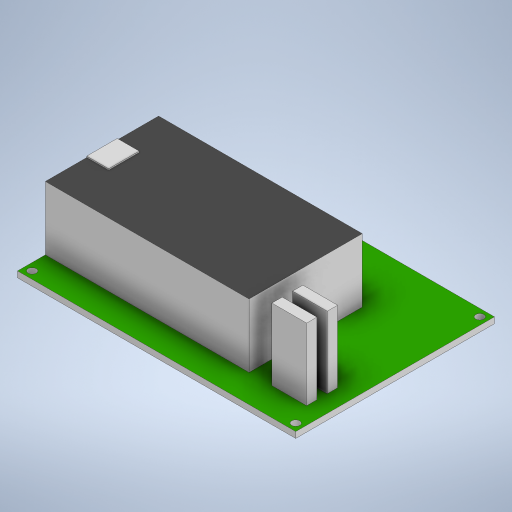
# Autodesk Inventor part: PCBModel
Saved by Autodesk Inventor 2024 (Build 280153000, 153)
## iProperties
Created: 2024-05-21
Part Number: PCBModel
Material: Generic
Document SubType Name: Modeling
Designer: andre
Density: 1 g/cm^3
Appearance: Default
Author: andre
Autodesk Inventor part; units mm, degrees
ref_plane "YZ Plane" through (0, 0, 0) normal (1, 0, 0) x (0, 1, 0)
ref_plane "XZ Plane" through (0, 0, 0) normal (0, 1, 0) x (-1, 0, 0)
ref_plane "XY Plane" through (0, 0, 0) normal (0, 0, 1) x (1, 0, 0)
sketch "Sketch1" plane through (0, 0, 0) normal (0, 1, 0) x (-1, 0, 0)
  line L0 (-35, 25) -> (35, 25)
  line L1 (35, 25) -> (35, -25)
  line L2 (35, -25) -> (-35, -25)
  line L3 (-35, -25) -> (-35, 25)
  line L4 (-35, 25) -> (35, -25) construction
  line L5 (35, 25) -> (-35, -25) construction
  point P0 (0, 0)
  dimension "d0" = 70
  dimension "d1" = 50
  constraints: 12 end point, 2 midpoint, 2 parallel, 1 horizontal, 1 perpendicular
  measures "d0" distance of L1.end L2.end
  measures "d1" distance of L0.end L1.end
extrude "Extrusion1" add sketch "Sketch1" along normal blind 1.5
sketch "Sketch4" plane through (0, 1.5, 0) normal (0, 1, 0) x (1, 0, 0)
  line L0 (16.25, 10.5) -> (-35, 10.5)
  line L1 (-35, 10.5) -> (-35, -18)
  line L2 (-35, -18) -> (16.25, -18)
  line L3 (16.25, -18) -> (16.25, 10.5)
  line L4 (16.25, 10.5) -> (-35, -18) construction
  line L5 (-35, 10.5) -> (16.25, -18) construction
  line L6 (-35, -25) -> (35, -25) projected
  line L7 (-35, 25) -> (-35, -25) projected
  dimension "d10" = 51.25
  dimension "d11" = 28.5
  dimension "d12" = 7
  constraints: 12 end point, 2 parallel, 1 collinear, 1 horizontal, 1 perpendicular
  measures "d10" distance of L2.end L1.end
  measures "d11" distance of L1.end L0.end
  measures "d12" distance between parallel lines of L6 L2
extrude "Extrusion3" add sketch "Sketch4" along normal blind 16
sketch "Sketch5" plane through (0, 1.5, 0) normal (0, 1, 0) x (1, 0, 0)
  line L0 (30.74, -15.4) -> (22, -15.4)
  line L1 (22, -15.4) -> (22, -18)
  line L2 (22, -18) -> (30.74, -18)
  line L3 (30.74, -18) -> (30.74, -15.4)
  line L4 (30.74, -15.4) -> (22, -18) construction
  line L5 (22, -15.4) -> (30.74, -18) construction
  line L6 (16.25, -18) -> (16.25, 10.5) projected
  line L7 (-35, -18) -> (16.25, -18) projected
  line L8 (30.74, -10.2) -> (22, -10.2)
  line L9 (22, -10.2) -> (22, -12.8)
  line L10 (22, -12.8) -> (30.74, -12.8)
  line L11 (30.74, -12.8) -> (30.74, -10.2)
  line L12 (30.74, -10.2) -> (22, -12.8) construction
  line L13 (22, -10.2) -> (30.74, -12.8) construction
  point P0 (0, 0)
  point P1 (26.37, -16.7)
  point P2 (22, -16.7)
  point P3 (26.37, -11.5)
  point P4 (22, -11.5)
  dimension "d15" = 5.75
  dimension "d16" = 8.74
  dimension "d17" = 2.6
  dimension "d18" = 8.74
  dimension "d19" = 2.6
  dimension "d20" = 2.6
  constraints: 24 end point, 6 midpoint, 4 parallel, 2 horizontal, 2 perpendicular, 1 collinear
  measures "d15" distance from line of L6 point (22, -16.7)
  measures "d16" distance of L1.end L2.end
  measures "d17" distance of L2.end L0.start
  measures "d18" distance of L9.end L10.end
  measures "d19" distance of L10.end L8.start
  measures "d20" distance between parallel lines of L0 L10
extrude "Extrusion4" add sketch "Sketch5" along normal blind 18
sketch "Sketch6" plane through (-35, 0, -25) normal (-1, 0, 0) x (0, 0, 1)
  line L0 (24.91, 17.82) -> (32.59, 17.82)
  line L1 (32.59, 17.82) -> (32.59, 15.11)
  line L2 (32.59, 15.11) -> (24.91, 15.11)
  line L3 (24.91, 15.11) -> (24.91, 17.82)
  line L4 (24.91, 17.82) -> (32.59, 15.11) construction
  line L5 (32.59, 17.82) -> (24.91, 15.11) construction
  line L6 (43, 1.5) -> (50, 1.5) projected
  line L7 (43, 1.5) -> (43, 17.5) projected
  line L8 (14.5, 1.5) -> (14.5, 17.5) projected
  line L9 (32.18, 17.41) -> (25.32, 17.41)
  line L10 (25.32, 17.41) -> (25.32, 15.52)
  line L11 (25.32, 15.52) -> (32.18, 15.52)
  line L12 (32.18, 15.52) -> (32.18, 17.41)
  point P0 (25, 0)
  point P1 (28.75, 16.465)
  dimension "d23" = 16.32
  dimension "d24" = 2.71
  dimension "d25" = 7.68
  dimension "d26" = 14.25
  dimension "d27" = 14.25
  dimension "d28" = 0.41
  constraints: 20 end point, 4 parallel, 2 midpoint, 2 perpendicular, 1 horizontal, 3 other
  measures "d23" distance between parallel lines of L6 L0
  measures "d24" distance between parallel lines of L0 L2
  measures "d25" distance between parallel lines of L3 L1
  measures "d26" distance from line of point (28.75, 16.465) L7
  measures "d27" distance from line of L8 point (28.75, 16.465)
  measures "d28" distance between parallel lines of L0 L9
extrude "Extrusion5" add sketch "Sketch6" against normal blind 5.51
sketch "Sketch7" plane through (-35, 0, -25) normal (-1, 0, 0) x (0, 0, 1)
  line L0 (32.18, 17.41) -> (25.32, 17.41) projected
  line L1 (25.32, 17.41) -> (25.32, 15.52) projected
  line L2 (25.32, 15.52) -> (32.18, 15.52) projected
  line L3 (32.18, 15.52) -> (32.18, 17.41) projected
  point P0 (25, 0)
extrude "Extrusion6" cut sketch "Sketch7" against normal blind 4.99
sketch "Sketch8" plane through (0, 1.5, 0) normal (0, 1, 0) x (1, 0, 0)
  circle A0 centre (33.16, -23.16) radius 1
  circle A1 centre (-33.16, -23.16) radius 1
  circle A2 centre (-33.16, 23.16) radius 1
  circle A3 centre (33.16, 23.16) radius 1
  line L0 (22, -10.2) -> (30.74, -10.2) projected
  line L1 (30.74, -10.2) -> (30.74, -12.8) projected
  line L2 (30.74, -12.8) -> (22, -12.8) projected
  line L3 (22, -12.8) -> (22, -10.2) projected
  line L4 (22, -15.4) -> (30.74, -15.4) projected
  line L5 (30.74, -15.4) -> (30.74, -18) projected
  line L6 (30.74, -18) -> (22, -18) projected
  line L7 (22, -18) -> (22, -15.4) projected
  line L8 (16.25, -18) -> (-35, -18) projected
  line L9 (-35, -18) -> (-35, -25) projected
  line L10 (-35, -25) -> (35, -25) projected
  line L11 (35, -25) -> (35, 25) projected
  line L12 (35, 25) -> (-35, 25) projected
  line L13 (-35, 25) -> (-35, 10.5) projected
  line L14 (-35, 10.5) -> (16.25, 10.5) projected
  line L15 (16.25, 10.5) -> (16.25, -18) projected
  point P0 (0, 0)
  dimension "d33" = 2
  dimension "d34" = 2
  dimension "d35" = 2
  dimension "d36" = 2
  dimension "d37" = 1.84
  dimension "d38" = 1.84
  dimension "d39" = 1.84
  dimension "d40" = 1.84
  dimension "d41" = 1.84
  dimension "d42" = 1.84
  dimension "d43" = 1.84
  dimension "d44" = 1.84
  constraints: 4 centre point
  measures "d33" diameter of A0
  measures "d34" diameter of A1
  measures "d35" diameter of A2
  measures "d36" diameter of A3
  measures "d37" distance from line of L10 A1.centre
  measures "d38" distance from line of L9 A1.centre
  measures "d39" distance from line of L11 A0.centre
  measures "d40" distance from line of L10 A0.centre
  measures "d41" distance from line of L11 A3.centre
  measures "d42" distance from line of L12 A3.centre
  measures "d43" distance from line of L12 A2.centre
  measures "d44" distance from line of L13 A2.centre
extrude "Extrusion7" cut sketch "Sketch8" against normal blind 10 contours A0 | A1 | A2 | A3
equation "\"d26\" = d27"
equation "\"d38\" = d37"
equation "\"d39\" = d37"
equation "\"d40\" = d37"
equation "\"d41\" = d37"
equation "\"d42\" = d37"
equation "\"d43\" = d37"
equation "\"d44\" = d37"
body "Solid1"
